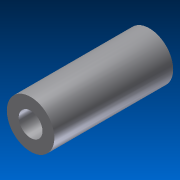
# Autodesk Inventor part: separador15
Saved by Autodesk Inventor 2012 (Build 160160000, 160)
## iProperties
Created: 2016-01-04
Part Number: separador15
Material: Default
Document SubType Name: Modeling
Designer: Alex Becerra
Mass: 0.318086 g
Surface Area: 4.66527 cm^2
Volume: 0.318086 cm^3
Density: 1 g/cm^3
Author: Alex Becerra
Autodesk Inventor part; units mm, degrees
ref_plane "YZ Plane" through (0, 0, 0) normal (1, 0, 0) x (0, 1, 0)
ref_plane "XZ Plane" through (0, 0, 0) normal (0, 1, 0) x (-1, 0, 0)
ref_plane "XY Plane" through (0, 0, 0) normal (0, 0, 1) x (1, 0, 0)
sketch "Sketch1" plane through (0, 0, 0) normal (0, 0, 1) x (1, 0, 0)
  circle A0 centre (0, 0) radius 1.5
  circle A1 centre (0, 0) radius 3
  dimension "d0" = 3
  dimension "d1" = 6
  constraints: 2 centre point, 2 coincident
  measures "d0" diameter of A0
  measures "d1" diameter of A1
extrude "Extrusion1" add sketch "Sketch1" along normal blind 15
body "Solid1"
